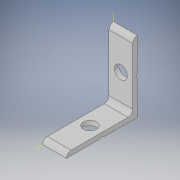
# Autodesk Inventor part: BTwinkel1_trajan20_21
Saved by Autodesk Inventor 2022.2 (Build 262287000, 287)
## iProperties
Company: HTBLA Kaindorf
RuleStatus: InUse
Created: 2022-06-22
Part Number: BTwinkel1_trajan20_21
Project: Zeichenmaschine_v2
Material: Generisch
Description: profil
Document SubType Name: Modeling
Designer: trajan20
Density: 1 g/cm^3
Appearance: Vorgabe
Mass: 1.05128 g
Surface Area: 13.7978 cm^2
Volume: 1.05128 cm^3
AfterDocNew0: iProperties-Editor_aufrufen
Author: jan
Keywords: 2021
Autodesk Inventor part; units mm, degrees
ref_plane "YZ Plane" through (0, 0, 0) normal (1, 0, 0) x (0, 1, 0)
ref_plane "XZ Plane" through (0, 0, 0) normal (0, 1, 0) x (-1, 0, 0)
ref_plane "XY Plane" through (0, 0, 0) normal (0, 0, 1) x (1, 0, 0)
sketch "Skizze4" plane through (0, 0, 0) normal (0, 1, 0) x (-1, 0, 0)
  line L0 (0, 0) -> (-30, 0)
  line L1 (-14.25, 0) -> (-15, 0.75)
  line L2 (-15, 0.75) -> (-15.75, 0)
  line L3 (-4, 2) -> (-28, 2)
  arc A0 (-28, 2) -> (-30, 0) centre (-28, 0) ccw
  circle A1 centre (-4, 4) radius 2
  line L4 (0, -8) -> (0, 48) projected
  line L5 (6.0828, 0) -> (-36.4971, 0) projected
  line L6 (0, 0) -> (-2.5858, 2.5858)
  point P0 (0, 40)
  dimension "d20" = 4
  dimension "d4" = 30
  dimension "d5" = 40
  dimension "d6" = 135
  dimension "d8" = 0.75
  dimension "d13" = 2
  dimension "d14" = 2
  dimension "d21" = 2
  dimension "d47" = 45
  dimension "d48" = 14.25
  dimension "d49" = 4
  constraints: 10 end point, 3 point on line, 2 horizontal, 2 point on circle, 1 centre point, 1 perpendicular, 3 other
  measures "d4" distance of L0.start L0.end
  measures "d5" distance of L0.start point (0, 40)
  measures "d6" angle of L0 L1
  measures "d8" horizontal distance of L2.end L1.end
  measures "d13" distance between parallel lines of L0 L3
  measures "d14" horizontal distance of L0.end L3.end
  measures "d21" distance from line of L3 point (-4, 4)
  measures "d47" angle of L5 L6
  measures "d48" distance from line of L4 L1.start
  measures "d49" distance from line of L4 point (-4, 4)
extrude "Extrusion3" add sketch "Skizze4" along normal blind 10 contours L0 L1 L2 A0 L3 A1 L6
sketch "Skizze6" plane through (4, 0, 2) normal (0, 0, 1) x (1, 0, 0)
  line L0 (0, 10) -> (24, 10) projected
  line L1 (0, 0) -> (24, 0) projected
  line L2 (26, 0) -> (26, 10) projected
  line L3 (-4, 0) -> (-4, 10) projected
  point P0 (11, 5)
  dimension "d37" = 10
  dimension "d38" = 5
  dimension "d39" = 15
  dimension "d50" = 30
  measures "d37" distance between parallel lines of L0 L1
  measures "d38" distance from line of L0 point (11, 5)
  measures "d39" distance from line of L2 point (11, 5)
  measures "d50" distance between parallel lines of L3 L2
hole "Bohrung2" at (15, 5, 2) direction (0, 0, -1) diameter 5.5 end through all
mirror "Spiegeln1" about plane through (0, 0, 0) normal (-0.7071068, 0, 0.7071068)
equation "\"d48\" = 0.5 * d4 - d8"
equation "\"d38\" = 0.5 * d37"
equation "\"d39\" = 0.5 * d50"
